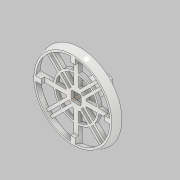
# Autodesk Inventor part: TopConnector
Saved by Autodesk Inventor 2019.2 (Build 232265000, 265)
## iProperties
Created: 2019-01-29
Part Number: TopConnector
Material: ABS-Kunststoff
Document SubType Name: Modeling
Designer: Lion
Density: 1.06 g/cm^3
Appearance: Weiß
Mass: 39.1412 g
Surface Area: 325.573 cm^2
Volume: 36.9256 cm^3
Author: Lion
## iProperties of the stored document TopConnector_3D-Druck.ipt
Created: 2019-04-11
Part Number: TopConnector_3D-Druck
Material: Generisch
Document SubType Name: Modeling
Designer: Lion
Density: 1 g/cm^3
Appearance: Vorgabe
Author: Lion
Autodesk Inventor part; units mm, degrees
ref_plane "YZ Plane" through (0, 0, 0) normal (1, 0, 0) x (0, 1, 0)
ref_plane "XZ Plane" through (0, 0, 0) normal (0, 1, 0) x (-1, 0, 0)
ref_plane "XY Plane" through (0, 0, 0) normal (0, 0, 1) x (1, 0, 0)
derived "BaseTop.ipt"
sketch "Skizze2" plane through (0, 0, 0) normal (0, 0, 1) x (1, 0, 0)
  line L0 (-16, -6) -> (16, -6)
  line L1 (16, -6) -> (16, 6)
  line L2 (16, 6) -> (-16, 6)
  line L3 (-16, 6) -> (-16, -6)
  line L4 (-16, -6) -> (16, 6) construction
  line L5 (16, -6) -> (-16, 6) construction
  line L6 (-11, 6) -> (3, 6)
  line L7 (3, 6) -> (3, -6)
  line L8 (3, -6) -> (-11, -6)
  line L9 (-11, -6) -> (-11, 6)
  circle A0 centre (-13.5, 0) radius 1
  line L10 (-11, -6) -> (-16, 6) construction
  line L11 (-16, -6) -> (-11, 6) construction
  line L12 (0, 6) -> (0, -6) construction
  circle A1 centre (13.5, 0) radius 1
  line L13 (-16, -26) -> (-16, 6)
  line L14 (-16, 6) -> (-28, 6)
  line L15 (-28, 6) -> (-28, -26)
  line L16 (-28, -26) -> (-16, -26)
  line L17 (-16, -26) -> (-28, 6) construction
  line L18 (-16, 6) -> (-28, -26) construction
  line L19 (-28, -21) -> (-28, -7)
  line L20 (-28, -7) -> (-16, -7)
  line L21 (-16, -7) -> (-16, -21)
  line L22 (-16, -21) -> (-28, -21)
  circle A2 centre (-22, -23.5) radius 1
  line L23 (-16, -21) -> (-28, -26) construction
  line L24 (-16, -26) -> (-28, -21) construction
  line L25 (-28, -10) -> (-16, -10) construction
  circle A3 centre (-22, 3.5) radius 1
  line L26 (-1, -26) -> (4, -38) construction
  line L27 (-15, -38) -> (-15, -26)
  line L28 (-12, -38) -> (-12, -26) construction
  line L29 (4, -26) -> (-28, -26)
  line L30 (-28, -38) -> (4, -38)
  line L31 (4, -26) -> (-28, -38) construction
  line L32 (-28, -26) -> (4, -38) construction
  line L33 (-1, -26) -> (-1, -38)
  line L34 (-15, -26) -> (-1, -26)
  line L35 (4, -26) -> (-1, -38) construction
  line L36 (4, -38) -> (4, -26)
  circle A4 centre (1.5, -32) radius 1
  line L37 (-1, -38) -> (-15, -38)
  circle A5 centre (-25.5, -32) radius 1
  line L38 (-28, -26) -> (-28, -38)
  line L39 (4, -11) -> (16, -6) construction
  line L40 (16, -25) -> (4, -25)
  line L41 (16, -22) -> (4, -22) construction
  line L42 (4, -6) -> (4, -38)
  line L43 (16, -38) -> (16, -6)
  line L44 (4, -6) -> (16, -38) construction
  line L45 (4, -38) -> (16, -6) construction
  line L46 (4, -11) -> (16, -11)
  line L47 (4, -25) -> (4, -11)
  line L48 (4, -6) -> (16, -11) construction
  line L49 (16, -6) -> (4, -6)
  circle A6 centre (10, -8.5) radius 1
  line L50 (16, -11) -> (16, -25)
  circle A7 centre (10, -35.5) radius 1
  line L51 (4, -38) -> (16, -38)
  line L52 (-16, -26) -> (4, -6) construction
  line L53 (4, -26) -> (-16, -6) construction
  line L54 (1, -23) -> (-13, -23)
  line L55 (-13, -23) -> (-13, -9)
  line L56 (-13, -9) -> (1, -9)
  line L57 (1, -9) -> (1, -23)
  line L58 (1, -23) -> (-13, -9) construction
  line L59 (-13, -23) -> (1, -9) construction
  line L60 (4, -25) -> (16, -25)
  line L61 (16, -25) -> (16, -38)
  line L62 (16, -38) -> (4, -38)
  line L63 (4, -38) -> (4, -25)
  line L64 (-13, -23) -> (1, -23)
  line L65 (1, -23) -> (1, -9)
  line L66 (1, -9) -> (-13, -9)
  line L67 (-13, -9) -> (-13, -23)
  line L68 (-13, -23) -> (1, -9) construction
  line L69 (1, -23) -> (-13, -9) construction
  line L70 (4, -6) -> (4, -26)
  line L71 (-16, -26) -> (4, -26)
  line L72 (4, -6) -> (-16, -6)
  line L73 (-16, -26) -> (-16, -6)
  point P0 (0, 0)
  point P1 (-13.5, 0)
  point P2 (-22, -10)
  point P3 (-12, -32)
  point P4 (10, -22)
  point P5 (-6, -16)
  dimension "d11" = 3
  measures "d11" distance between parallel lines of L42 L65
extrude "Extrusion3" add sketch "Skizze2" along normal blind 3 contours L0 L42 L29 L13
sketch "Skizze3" plane through (-13, -23, 3) normal (0, 0, 1) x (1, 0, 0)
  line L0 (-3, -3) -> (17, -3) projected
  line L1 (17, -3) -> (17, 17) projected
  line L2 (17, 17) -> (-3, 17) projected
  line L3 (-3, 17) -> (-3, -3) projected
  line L4 (17, -3) -> (-3, 17) construction
  line L5 (17, 17) -> (-3, -3) construction
  line L6 (15.5, 15.5) -> (-1.5, 15.5)
  line L7 (-1.5, 15.5) -> (-1.5, -1.5)
  line L8 (-1.5, -1.5) -> (15.5, -1.5)
  line L9 (15.5, -1.5) -> (15.5, 15.5)
  line L10 (15.5, 15.5) -> (-1.5, -1.5) construction
  line L11 (-1.5, 15.5) -> (15.5, -1.5) construction
  point P0 (7, 7)
  dimension "d14" = 1.5
  constraints: 16 end point, 3 midpoint, 2 parallel, 2 perpendicular, 1 horizontal, 1 point on line
  measures "d14" distance between parallel lines of L0 L8
extrude "Extrusion2" add sketch "Skizze3" along normal blind 35
chamfer "Fase2" distance 2.8 angle 45 8 edges at (4, -26, 19) (4, -6, 19) (-16, -26, 19) (-16, -6, 19) (-14.5, -7.5, 20.5) (2.5, -7.5, 20.5) (2.5, -24.5, 20.5) (-14.5, -24.5, 20.5)
fillet "Rundung1" radius 2 4 edges at (-13, -9, 1.5) (1, -9, 1.5) (1, -23, 1.5) (-13, -23, 1.5)
derived "ShellLower.ipt"
sketch "Skizze6" plane through (-13, -23, 38) normal (0, 0, 1) x (1, 0, 0)
  line L0 (14.2, 17) -> (-0.2, 17) construction
  line L1 (-3, 14.2) -> (-3, -0.2) construction
  line L2 (-0.2, -3) -> (14.2, -3) construction
  line L3 (17, -0.2) -> (17, 14.2) construction
  line L4 (-3, -3) -> (17, -3) construction
  line L5 (17, -3) -> (17, 17) construction
  line L6 (17, 17) -> (-3, 17) construction
  line L7 (-3, 17) -> (-3, -3) construction
  line L8 (-3, -3) -> (17, 17) construction
  line L9 (17, -3) -> (-3, 17) construction
  circle A0 centre (7, 7) radius 60
  circle A1 centre (7, 7) radius 62.5
  line L10 (3.5, -52.8978) -> (10.5, -52.8978)
  line L11 (10.5, -52.8978) -> (10.5, 66.8978)
  line L12 (10.5, 66.8978) -> (3.5, 66.8978)
  line L13 (3.5, 66.8978) -> (3.5, -52.8978)
  line L14 (3.5, -52.8978) -> (10.5, 66.8978) construction
  line L15 (10.5, -52.8978) -> (3.5, 66.8978) construction
  line L16 (-52.8978, 10.5) -> (66.8978, 10.5)
  line L17 (66.8978, 10.5) -> (66.8978, 3.5)
  line L18 (66.8978, 3.5) -> (-52.8978, 3.5)
  line L19 (-52.8978, 3.5) -> (-52.8978, 10.5)
  line L20 (-52.8978, 10.5) -> (66.8978, 3.5) construction
  line L21 (66.8978, 10.5) -> (-52.8978, 3.5) construction
  line L22 (-0.2, 17) -> (17, -0.2) construction
  line L23 (8.4, 8.4) -> (11.2284, 11.2284)
  line L24 (11.2284, 11.2284) -> (-32.763, 55.2199)
  line L25 (-32.763, 55.2199) -> (-35.5914, 52.3914)
  line L26 (-35.5914, 52.3914) -> (8.4, 8.4)
  line L27 (2.7716, 11.2284) -> (-41.2199, -32.763)
  line L28 (-41.2199, -32.763) -> (-38.3914, -35.5914)
  line L29 (-38.3914, -35.5914) -> (5.6, 8.4)
  line L30 (5.6, 8.4) -> (2.7716, 11.2284)
  line L31 (2.7716, 2.7716) -> (46.763, -41.2199)
  line L32 (46.763, -41.2199) -> (49.5914, -38.3914)
  line L33 (49.5914, -38.3914) -> (5.6, 5.6)
  line L34 (5.6, 5.6) -> (2.7716, 2.7716)
  line L35 (11.2284, 2.7716) -> (55.2199, 46.763)
  line L36 (55.2199, 46.763) -> (52.3914, 49.5914)
  line L37 (52.3914, 49.5914) -> (8.4, 5.6)
  line L38 (8.4, 5.6) -> (11.2284, 2.7716)
  line L39 (-3, -0.2) -> (-0.2, -3) construction
  line L40 (14.2, 17) -> (-3, -0.2) construction
  line L41 (5.6, 8.4) -> (2.7716, 11.2284)
  line L42 (2.7716, 11.2284) -> (46.763, 55.2199)
  line L43 (46.763, 55.2199) -> (49.5914, 52.3914)
  line L44 (49.5914, 52.3914) -> (5.6, 8.4)
  line L45 (-38.3914, 49.5914) -> (5.6, 5.6)
  line L46 (2.7716, 2.7716) -> (-41.2199, 46.763)
  line L47 (5.6, 5.6) -> (2.7716, 2.7716)
  line L48 (-41.2199, 46.763) -> (-38.3914, 49.5914)
  line L49 (-35.5914, -38.3914) -> (8.4, 5.6)
  line L50 (11.2284, 2.7716) -> (-32.763, -41.2199)
  line L51 (8.4, 5.6) -> (11.2284, 2.7716)
  line L52 (-32.763, -41.2199) -> (-35.5914, -38.3914)
  line L53 (52.3914, -35.5914) -> (8.4, 8.4)
  line L54 (11.2284, 11.2284) -> (55.2199, -32.763)
  line L55 (8.4, 8.4) -> (11.2284, 11.2284)
  line L56 (55.2199, -32.763) -> (52.3914, -35.5914)
  circle A2 centre (7, 7) radius 30
  circle A3 centre (7, 7) radius 33
  point P0 (13, 23)
  dimension "d30" = 120
  dimension "d31" = 2.5
  dimension "d32" = 7
  dimension "d33" = 7
  dimension "d35" = 4
  dimension "d38" = 360
  dimension "d42" = 360
  dimension "d44" = 60
  dimension "d45" = 3
  constraints: 104 end point, 11 parallel, 7 midpoint, 6 perpendicular, 5 collinear, 4 centre point, 4 coincident, 4 point on circle, 3 horizontal, 3 point on line, 66 other
  measures "d30" diameter of A0
  measures "d31" radial gap between concentric circles of A1 A0
  measures "d32" distance between parallel lines of L11 L13
  measures "d33" distance between parallel lines of L18 L16
  measures "d35" distance between parallel lines of L26 L24
  measures "d44" diameter of A2
  measures "d45" radial gap between concentric circles of A2 A3
extrude "Extrusion5" add sketch "Skizze6" along normal blind 5 contours L17 L18 A3 L16 | L35 A3 L37 A0 | A0 L37 L36 L35 | A3 L18 A2 L16 | L16 A2 L35 A3 | L54 L56 L53 A0 | A0 L53 A3 L54 | A3 L54 A2 L18 | L35 A2 L37 A3 | A2 L18 L54 L35 L16 | A3 L53 A2 L54 | L44 A3 L42 A0 | A0 L42 L43 L44 | L37 A2 L44 A3 | L35 L16 L37 A2 | L35 L54 L37 L16 | L33 L32 L31 A0 | A0 L31 A3 L33 | A3 L33 A2 L53 | A2 L53 L18 L54 | L18 L53 L35 L54 | L44 A2 L42 A3 | L24 A0 L26 L25 | L37 L54 L16 | L35 L53 L11 L37 L54 | A3 L31 A2 L33 | L52 L49 A0 L50 | L18 L35 L53 | L11 A3 L13 L12 | L42 A2 L11 A3 | L44 L11 L42 A2 | L48 L45 A0 L46 | L24 A3 L26 A0 | L54 L37 L11 L16 | L16 L23 L54 | L35 L18 L11 L53 | L10 L13 A3 L11 | A3 L11 A2 L31 | A2 L31 L11 L33 | L27 A0 L29 L28 | A0 L49 A3 L50 | L35 L38 L18 | L11 A2 L13 A3 | L44 L24 L42 L11 | L11 L24 L44 | A0 L45 A3 L46 | A3 L13 A2 L24 | L24 A2 L26 A3 | L16 L44 L24 L11 | L23 L26 L44 L16 | L11 L37 L53 L23 | L11 L24 L23 | L11 L53 L37 | L11 L38 L37 L53 | A3 L13 A2 L11 | L33 L50 L11 | L11 L31 L50 L33 | L27 A3 L29 A0 | A3 L49 A2 L50 | L50 A2 L13 A3 | L38 L50 L11 | L11 L50 L33 L18 | L18 L33 L49 L38 | L11 L42 L24 L13 A2 | L44 L16 L26 L42 L24 | L16 A3 L18 L19 | A3 L45 A2 L46 | L46 A2 L16 A3 | L26 A2 L45 A3 | L24 L13 L26 A2 | L44 L26 L16 | L53 L37 L49 L33 L45 L29 L44 L26 | A2 L13 L50 L31 L11 | L50 L31 L49 L18 L33 | A3 L18 A2 L27 | L27 A2 L29 A3 | A3 L29 A2 L49 | A2 L49 L13 L50 | L18 L49 L33 | L42 L26 L13 L24 | L16 A2 L18 A3 | A2 L45 L16 L46 | L26 L44 L30 L16 | L16 L13 L42 L26 | L50 L13 L49 L31 | L27 L18 L29 A2 | L49 L31 L13 L18 | L18 L34 L33 L49 | L42 L13 L26 | L16 L46 L27 L18 A2 | L16 L45 L27 L46 | L30 L42 L13 | L30 L29 L45 L13 | L13 L45 L27 L16 | L16 L27 L30 | L49 L13 L31 | L27 L46 L29 L18 | L18 L46 L29 L13 | L34 L46 L18 | L13 L29 L45 L34 | L13 L31 L34 | L16 L27 L45 | L27 L45 L13 L29 L46 | L45 L29 L13 | L29 L46 L18
sketch "Skizze7" plane through (-13, -23, 43) normal (0, 0, 1) x (1, 0, 0)
  line L0 (-0.2, 17) -> (-3, 14.2) projected
  line L1 (14.2, 17) -> (-0.2, 17) projected
  line L2 (17, 14.2) -> (14.2, 17) projected
  line L3 (17, -0.2) -> (17, 14.2) projected
  line L4 (14.2, -3) -> (17, -0.2) projected
  line L5 (-0.2, -3) -> (14.2, -3) projected
  line L6 (-3, -0.2) -> (-0.2, -3) projected
  line L7 (-3, 14.2) -> (-3, -0.2) projected
  line L8 (0, 12) -> (0, 2) projected
  arc A0 (0, 2) -> (2, 0) centre (2, 2) ccw projected
  line L9 (2, 0) -> (12, 0) projected
  arc A1 (12, 0) -> (14, 2) centre (12, 2) ccw projected
  line L10 (14, 2) -> (14, 12) projected
  arc A2 (14, 12) -> (12, 14) centre (12, 12) ccw projected
  line L11 (12, 14) -> (2, 14) projected
  arc A3 (2, 14) -> (0, 12) centre (2, 12) ccw projected
  point P0 (13, 23)
extrude "Extrusion6" add sketch "Skizze7" against normal up to surface (5 mm away)
extrude "Extrusion7" cut sketch "Skizze7" against normal up to surface (5 mm away) contours A3 L11 A2 L10 A1 L9 A0 L8
chamfer "Fase3" distance 3 angle 45 8 edges at (-2.5, -4.0431, 40.5) (-9.5, -4.0431, 40.5) (-17.9569, -12.5, 40.5) (-17.9569, -19.5, 40.5) (-9.5, -27.9569, 40.5) (-2.5, -27.9569, 40.5) (5.9569, -19.5, 40.5) (5.9569, -12.5, 40.5)
chamfer "Fase4" distance 1 angle 45 4 edges at (-16, -16, 38) (-6, -26, 38) (4, -16, 38) (-6, -6, 38)
ref_plane "Arbeitsebene5" through (-13, -23, 22.5) normal (0, 0, 1) x (1, 0, 0)
sketch "Skizze8" plane through (-13, -23, 22.5) normal (0, 0, 1) x (1, 0, 0)
  arc A0 (66.75, 7) -> (-52.75, 7) centre (7, 7) ccw
  arc A1 (-55.25, 7) -> (69.25, 7) centre (7, 7) ccw construction
  line L0 (69.25, 7) -> (-55.25, 7)
  arc A2 (69.25, 7) -> (-55.25, 7) centre (7, 7) ccw
  arc A3 (-52.75, 7) -> (66.75, 7) centre (7, 7) ccw construction
  point P0 (13, 23)
  dimension "d59" = 119.5
  dimension "d60" = 2.5
  constraints: 8 point on circle, 4 centre point, 3 coincident, 2 end point, 2 point on line, 1 horizontal, 1 midpoint
  measures "d59" diameter of A0
  measures "d60" radial gap between concentric circles of A1 A0
revolve "Umdrehung2" add sketch "Skizze8" angle 180 about axis through (56.25, -16, 22.5) along (1, 0, 0) separate body contours A0 L0 A2
ref_plane "Arbeitsebene6" through (-13, -23, 37) normal (0, 0, 1) x (1, 0, 0)
split "Trennen3" plane through (-13, -23, 37) removes the side toward (0, 0, -1) bodies 2
ref_plane "Arbeitsebene7" through (-13, -23, 48) normal (0, 0, 1) x (1, 0, 0)
split "Trennen4" plane through (-13, -23, 48) removes the side toward (0, 0, 1) bodies 2
combine bodies "Kombinieren1" operation type add bodies to combine 2 1
delete faces "Fläche löschen1" heal yes whole lump no faces at (-52.3342, 25.6486, 39.6667) (-53.588, 23.1312, 40.2269) (-51.8171, 24.5021, 43) (-50.8225, 26.0225, 40.2269) (-52.174, 24.859, 38) (-46.7058, 31.277, 41.3333) (-45.1312, 31.588, 40.2269) (-46.859, 30.174, 38) (-46.5021, 29.8171, 43) (-48.0225, 28.8225, 40.2269) (-65.8978, -16.3914, 41.8032) (-65.2271, -12.5, 42.568) (-65.5206, -16.3891, 43) (-65.2271, -19.5, 42.568) (-52.3342, -57.6486, 39.6667) (-47.6486, -62.3342, 39.6667) (-51.8171, -56.5021, 43) (-46.5021, -61.8171, 43) (-48.0225, -60.8225, 40.2269) (-53.588, -55.1312, 40.2269) (-50.8225, -58.0225, 40.2269) (-45.1312, -63.588, 40.2269) (-5.6086, -75.8978, 41.8032) (-9.5, -75.2271, 42.568) (-5.6109, -75.5206, 43) (-2.5, -75.2271, 42.568) (35.6486, -62.3342, 41.3333) (34.5021, -61.8171, 43) (39.8171, -56.5021, 43) (40.3342, -57.6486, 39.6667) (33.1312, -63.588, 40.2269) (38.8225, -58.0225, 40.2269) (40.174, -56.859, 38) (34.859, -62.174, 38) (41.588, -55.1312, 40.2269) (36.0225, -60.8225, 40.2269) (53.8978, -16.3914, 41.8032) (53.2271, -12.5, 42.568) (53.5206, -16.3891, 43) (53.2271, -19.5, 42.568) (41.588, 23.1312, 40.2269) (40.3342, 25.6486, 41.3333) (39.8171, 24.5021, 43) (40.174, 24.859, 38) (34.859, 30.174, 38) (34.7058, 31.277, 39.6667) (34.5021, 29.8171, 43) (36.0225, 28.8225, 40.2269) (33.1312, 31.588, 40.2269) (38.8225, 26.0225, 40.2269) (-5.6086, 43.8978, 41.8032) (-5.6109, 43.5206, 43) (-2.5, 43.2271, 42.568) (-9.5, 43.2271, 42.568)
sketch "Skizze9" plane through (-62.0139, -12.5, 43) normal (0, 0, 1) x (1, 0, 0)
  arc A0 (59.5139, 52.5139) -> (52.5139, 52.5139) centre (56.0139, -3.5) ccw construction
  line L0 (59.5139, 29.3139) -> (59.5139, 52.5139) construction
  line L1 (52.5139, 52.5139) -> (52.5139, 29.3139) construction
  line L2 (59.5139, 42.6232) -> (52.5139, 42.6232)
  line L3 (52.5139, 42.6232) -> (52.5139, 52.6232)
  line L4 (52.5139, 52.6232) -> (59.5139, 52.6232)
  line L5 (59.5139, 52.6232) -> (59.5139, 42.6232)
  line L6 (9.8908, 0) -> (9.8908, -7)
  line L7 (9.8908, -7) -> (-0.1092, -7)
  line L8 (-0.1092, -7) -> (-0.1092, 0)
  line L9 (-0.1092, 0) -> (9.8908, 0)
  line L10 (52.5139, -49.6232) -> (59.5139, -49.6232)
  line L11 (59.5139, -49.6232) -> (59.5139, -59.6232)
  line L12 (59.5139, -59.6232) -> (52.5139, -59.6232)
  line L13 (52.5139, -59.6232) -> (52.5139, -49.6232)
  line L14 (102.1371, -7) -> (102.1371, 0)
  line L15 (102.1371, 0) -> (112.1371, 0)
  line L16 (112.1371, 0) -> (112.1371, -7)
  line L17 (112.1371, -7) -> (102.1371, -7)
  point P0 (62.0139, 12.5)
  point P1 (0, -7)
  point P2 (0, 0)
  point P3 (59.5139, -59.5139)
  point P4 (52.5139, -59.5139)
  point P5 (112.0279, 0)
  point P6 (112.0279, -7)
  dimension "d64" = 10
  dimension "d67" = 360
  constraints: 32 end point, 2 parallel, 2 point on line, 1 horizontal, 1 perpendicular, 1 tangent, 41 other
  measures "d64" distance between parallel lines of L2 L4
extrude "Extrusion8" add sketch "Skizze9" along normal up to surface (5 mm away) bodies 2
chamfer "Fase5" distance 1 angle 45 1 edges at (-6, -73.9639, 37)
fillet "Rundung2" [suppressed]
equation "\"d30\" = d_inner"
equation "\"d44\" = 0.5 * d_inner"
equation "\"foot_cut\" = -30.5"
equation "\"d_inner\" = 120"
